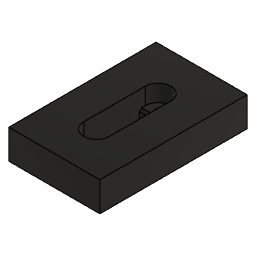
BottomPlateWithUSB (Autodesk Fusion 360 design; units mm, degrees)
Autodesk Fusion 360 part; units mm, degrees
sketch "Base Sketch" plane through (0, 0, 0) normal (0, 0, 1) x (1, 0, 0)
  line L0 (-19.62, 31.75) -> (19.62, 31.75)
  line L1 (19.62, 31.75) -> (19.62, -31.75)
  line L2 (19.62, -31.75) -> (-19.62, -31.75)
  line L3 (-19.62, -31.75) -> (-19.62, 31.75)
  line L4 (-19.62, 31.75) -> (19.62, -31.75) construction
  line L5 (19.62, 31.75) -> (-19.62, -31.75) construction
  dimension "d1" = 39.24
  dimension "d2" = 63.5
  constraint horizontal L0
  constraint perpendicular L0 L1
  constraint parallel L0 L2
  constraint parallel L1 L3
  constraint coincident L4 origin
  constraint coincident L5 origin
  measures "d1" distance of L0.start L0.end
  measures "d2" distance of L0.end L1.end
extrude "Plate Extrude" add sketch "Base Sketch" along normal blind 12.7
sketch "USB Slot Sketch" plane through (0, 0, 12.7) normal (0, 0, 1) x (-1, 0, 0)
  line L0 (19.62, 31.75) -> (-19.62, 31.75)
  line L1 (-19.62, 31.75) -> (-19.62, -31.75)
  line L2 (-19.62, -31.75) -> (19.62, -31.75)
  line L3 (19.62, -31.75) -> (19.62, 31.75)
  line L4 (-5.5, 13.5) -> (-5.5, -13)
  arc A0 (-5.5, -13) -> (5.5, -13) centre (0, -13) ccw
  line L5 (5.5, -13) -> (5.5, 13.5)
  arc A1 (5.5, 13.5) -> (-5.5, 13.5) centre (0, 13.5) ccw
  line L6 (0, 19) -> (0, -18.5) construction
  line L7 (0, -31.75) -> (0, 31.75) construction
  dimension "d5" = 11
  dimension "d6" = 13.25
  dimension "d8" = 37.5
  constraint tangent L4 A0
  constraint tangent A0 L5
  constraint parallel L4 L5
  constraint tangent L5 A1
  constraint tangent L4 A1
  constraint midpoint A1 L6.start
  constraint midpoint A0 L6.end
  constraint vertical L6
  constraint midpoint L2 L7.start
  constraint midpoint L0 L7.end
  constraint vertical L6.end L7.end
  measures "d5" diameter of A0
  measures "d6" distance of L2 L6.end
  measures "d8" distance of L6.start L6.end
extrude "Cut for USB (1)" cut sketch "USB Slot Sketch" against normal blind 7.25 contours L4 A0 L5 A1
sketch "USB Cavity Sketch" plane through (0, 0, 5.45) normal (0, 0, 1) x (-1, 0, 0)
  arc A0 (5.5, 13.5) -> (-5.5, 13.5) centre (0, 13.5) ccw
  line L0 (-5.5, 13.5) -> (-5.5, -13)
  arc A1 (-5.5, -13) -> (5.5, -13) centre (0, -13) ccw
  line L1 (5.5, -13) -> (5.5, 13.5)
  line L2 (5.5, -10.375) -> (-5.5, -10.375)
  line L3 (-5.5, -10.375) -> (-5.5, 10.375)
  line L4 (-5.5, 10.375) -> (5.5, 10.375)
  line L5 (5.5, 10.375) -> (5.5, -10.375)
  dimension "d11" = 20.75
  dimension "d12" = 10.375
  constraint horizontal L2
  constraint vertical L3
  constraint horizontal L4
  constraint vertical L5
  constraint coincident L0 L3.end
  constraint coincident L1 L2.start
  measures "d11" distance of L2 L4
  measures "d12" distance of origin L2
extrude "Cut for USB Back" cut sketch "USB Cavity Sketch" against normal blind 6 contours L0 L1 L2 L3 L4 L5
sketch "Screw Hole Sketch" plane through (0, 0, 5.45) normal (0, 0, 1) x (-1, 0, 0)
  line L0 (-5.5, 10.375) -> (5.5, 10.375)
  line L1 (5.5, 10.375) -> (5.5, 13.5)
  arc A0 (5.5, 13.5) -> (-5.5, 13.5) centre (0, 13.5) ccw
  line L2 (-5.5, 13.5) -> (-5.5, 10.375)
  circle A1 centre (0, 14.5) radius 2.1
  line L3 (0, 10.375) -> (0, 19) construction
  point P0 (0, 16.6)
  point P1 (0, 19)
  dimension "d16" = 2.4
  dimension "d17" = 4.2
  constraint coincident A1 P0
  constraint midpoint A0 P1
  constraint midpoint L0 L3.start
  constraint coincident P1 L3.end
  constraint vertical A1.centre L3.start
  measures "d16" distance of P0 P1
  measures "d17" diameter of A1
hole "Screw Hole" at (0, -14.5, 5.45) direction (0, 0, -1) diameter 3.332 depth 5 tip angle 180
mirror "Mirror Screw Hole" about plane through (0, 0, 0) normal (0, 1, 0) of "Screw Hole"
chamfer "Inner Chamfer" distance 1 angle 45 2 edges at (0, -10.375, 5.45) (0, 10.375, 5.45)
mesh "Mesh1" [no effect]
mesh "Mesh2" [no effect]
named bodies: "Bottom Plate"
